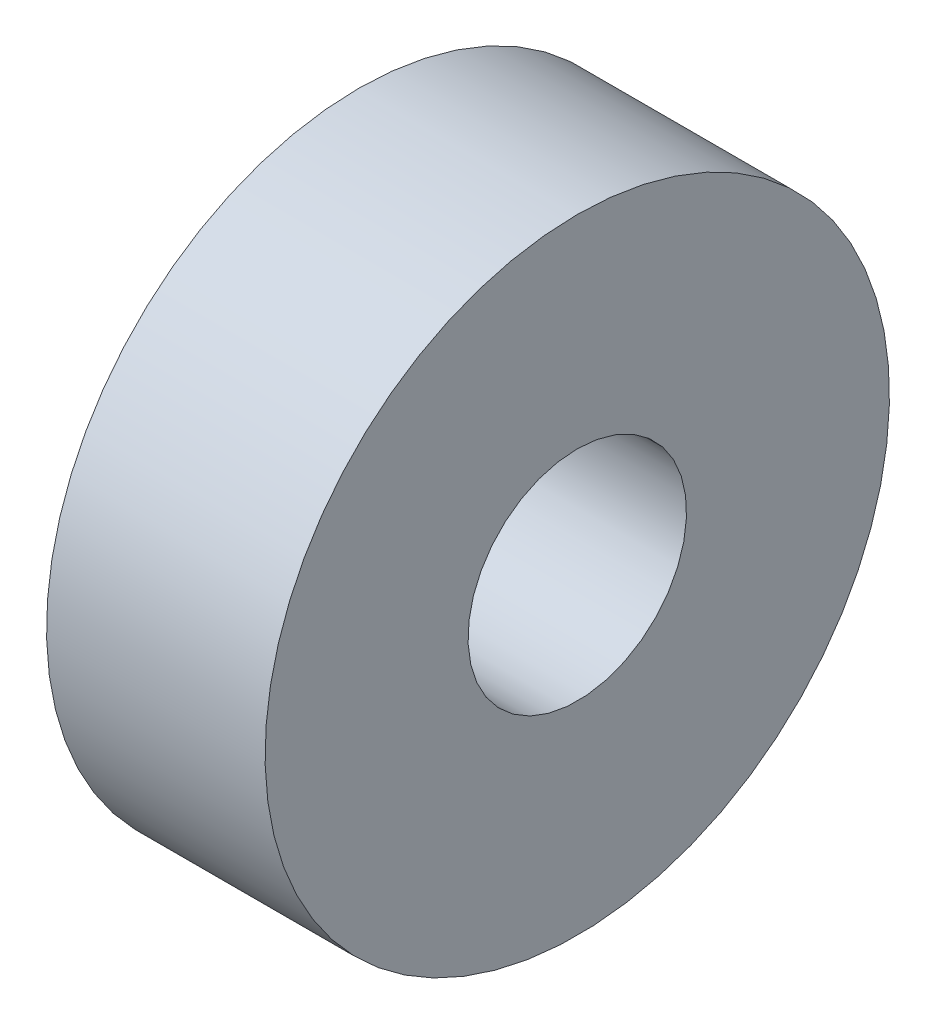
# Autodesk Inventor part: mtv_gear6_1-16
Saved by Autodesk Inventor 2018 (Build 220112000, 112)
## iProperties
Created: 2019-01-17
Part Number: mtv_gear6_1-16
Material: Generic
Document SubType Name: Modeling
Designer: aditya
Density: 1 g/cm^3
Appearance: Default
Author: aditya
Autodesk Inventor part; units mm, degrees
ref_plane "YZ Plane" through (0, 0, 0) normal (1, 0, 0) x (0, 1, 0)
ref_plane "XZ Plane" through (0, 0, 0) normal (0, 1, 0) x (-1, 0, 0)
ref_plane "XY Plane" through (0, 0, 0) normal (0, 0, 1) x (1, 0, 0)
sketch "Sketch1" plane through (0, 0, 0) normal (1, 0, 0) x (0, 1, 0)
  circle A0 centre (0, 0) radius 1.75
  circle A1 centre (0, 0) radius 5
  dimension "d0" = 3.5
  dimension "d1" = 10
  constraints: 2 centre point, 2 coincident
  measures "d0" diameter of A0
  measures "d1" diameter of A1
extrude "Extrusion1" add sketch "Sketch1" along normal blind 3.5
sketch "Sketch2" plane through (3.5, 0, 0) normal (1, 0, 0) x (0, 0, -1)
  circle A0 centre (0, 0) radius 5 construction
  line L0 (0, 5) -> (0, 4.5) construction
  line L1 (0, 4.5) -> (1, 4.5) construction
  line L2 (1, 4.5) -> (-1, 4.5) construction
  line L3 (0, 4.5) -> (0, 7.5) construction
  arc A1 (0, 7.5) -> (-1, 4.5) centre (2.4623, 5.0126) ccw
  line L4 (0, 7.5) -> (2, 7.5)
  dimension "d4" = 0.5
  dimension "d5" = 1
  dimension "d6" = 2
  dimension "d7" = 3
  dimension "d8" = 3.5
  dimension "d9" = 2
  constraints: 10 end point, 2 point on circle, 2 vertical, 1 centre point, 1 horizontal, 1 perpendicular, 1 point on line, 1 vertical alignment, 1 other
  measures "d4" distance of L0.start L0.end
  measures "d5" distance of L0.end L1.end
  measures "d6" distance of L1.end L2.end
  measures "d7" distance of L0.end L3.end
  measures "d8" radius of A1
  measures "d9" distance of L3.end L4.end
body "Solid1"
